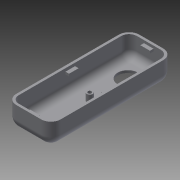
# Autodesk Inventor part: NodeMCU_MQ-7_top_shelled
Saved by Autodesk Inventor 2014 SP1 (Build 180222100, 222)
## iProperties
Created: 2016-10-27
Part Number: NodeMCU_MQ-7_top_shelled
Material: Generic
Document SubType Name: Modeling
Designer: danielsikar
Density: 1 g/cm^3
Appearance: Default
Author: danielsikar
Autodesk Inventor part; units mm, degrees
ref_plane "YZ Plane" through (0, 0, 0) normal (1, 0, 0) x (0, 1, 0)
ref_plane "XZ Plane" through (0, 0, 0) normal (0, 1, 0) x (-1, 0, 0)
ref_plane "XY Plane" through (0, 0, 0) normal (0, 0, 1) x (1, 0, 0)
sketch "Sketch1" plane through (0, 0, 0) normal (0, 0, 1) x (1, 0, 0)
  line L0 (0, 0) -> (37, 0)
  line L1 (37, 0) -> (37, 93.8)
  line L2 (28.5, 102.3) -> (8.5, 102.3)
  line L3 (0, 93.8) -> (0, 0)
  arc A0 (8.5, 102.3) -> (0, 93.8) centre (8.5, 93.8) ccw
  arc A1 (37, 93.8) -> (28.5, 102.3) centre (28.5, 93.8) ccw
  point P0 (37, 102.3)
  point P1 (0, 102.3)
  dimension "d0" = 37
  dimension "d1" = 102.3
  dimension "d11" = 8.5
  dimension "d12" = 8.5
  constraints: 8 end point, 4 point on circle, 4 point on line, 4 tangent, 2 centre point, 2 parallel, 1 horizontal, 1 perpendicular
  measures "d0" distance of point (0, 102.3) point (37, 102.3)
  measures "d1" distance of point (37, 102.3) L0.end
  measures "d11" radius of A0
  measures "d12" radius of A1
extrude "Extrusion1" add sketch "Sketch1" along normal blind 19
fillet "Fillet1" radius 8 2 edges at (0, 0, 9.5) (37, 0, 9.5)
fillet "Fillet2" radius 8 6 edges at (18.5, 102.3, 0) (0, 50.9, 0) (2.3431, 2.3431, 0) (18.5, 0, 0) (34.6569, 2.3431, 0) (37, 50.9, 0)
shell "Shell1" thickness 2 removed faces 1 at (12.3333, 36.6, 19)
sketch "Sketch2" plane through (0, 0, 0) normal (0, 0, -1) x (-1, 0, 0)
  circle A0 centre (-18.5, 82.8) radius 8.5
  line L0 (-8.5, 102.3) -> (-28.5, 102.3) projected
  point P0 (0, 0)
  point P1 (-8, 102.3)
  point P2 (-29, 102.3)
  dimension "d7" = 17
  dimension "d8" = 19.5
  constraints: 1 centre point
  measures "d7" diameter of A0
  measures "d8" distance from line of A0.centre L0
extrude "Extrusion2" cut sketch "Sketch2" against normal blind 19
sketch "Sketch3" plane through (8, 2, 8) normal (0, 1, 0) x (1, 0, 0)
  line L0 (21, -11) -> (0, -11) projected
  line L1 (6.6, -6.5) -> (14.6, -6.5)
  line L2 (14.6, -6.5) -> (14.6, -8.5)
  line L3 (14.6, -8.5) -> (6.6, -8.5)
  line L4 (6.6, -8.5) -> (6.6, -6.5)
  point P0 (-8, 8)
  point P1 (29, -11)
  dimension "d13" = 8
  dimension "d14" = 2
  dimension "d15" = 2.5
  dimension "d16" = 14.4
  constraints: 8 end point, 2 parallel, 1 horizontal, 1 perpendicular
  measures "d13" distance of L2.end L3.end
  measures "d14" distance of L1.end L2.end
  measures "d15" distance between parallel lines of L3 L0
  measures "d16" distance from line of point (29, -11) L2
extrude "Extrusion3" add sketch "Sketch3" along normal blind 3
sketch "Sketch4" plane through (2, 8, 8) normal (1, 0, 0) x (0, 0, -1)
  line L0 (-11, 0) -> (-11, 85.8) projected
  line L1 (-8.5, 47.15) -> (-6.5, 47.15)
  line L2 (-6.5, 47.15) -> (-6.5, 39.15)
  line L3 (-6.5, 39.15) -> (-8.5, 39.15)
  line L4 (-8.5, 39.15) -> (-8.5, 47.15)
  point P0 (8, -8)
  point P1 (-11, 94.3)
  dimension "d19" = 2
  dimension "d20" = 8
  dimension "d21" = 2.5
  dimension "d24" = 47.15
  constraints: 8 end point, 2 parallel, 1 horizontal, 1 perpendicular
  measures "d19" distance of L2.end L3.end
  measures "d20" distance of L1.end L2.end
  measures "d21" distance between parallel lines of L4 L0
  measures "d24" distance from line of point (-11, 94.3) L1
extrude "Extrusion4" add sketch "Sketch4" along normal blind 3
sketch "Sketch5" plane through (35, 8, 8) normal (-1, 0, 0) x (0, 0, 1)
  line L0 (11, 85.8) -> (11, 0) projected
  line L1 (6.5, 47.15) -> (8.5, 47.15)
  line L2 (8.5, 47.15) -> (8.5, 39.15)
  line L3 (8.5, 39.15) -> (6.5, 39.15)
  line L4 (6.5, 39.15) -> (6.5, 47.15)
  point P0 (-8, -8)
  point P1 (11, 94.3)
  dimension "d25" = 2
  dimension "d26" = 8
  dimension "d27" = 2.5
  dimension "d30" = 47.15
  constraints: 8 end point, 2 parallel, 1 horizontal, 1 perpendicular
  measures "d25" distance of L2.end L3.end
  measures "d26" distance of L1.end L2.end
  measures "d27" distance between parallel lines of L0 L2
  measures "d30" distance from line of point (11, 94.3) L1
extrude "Extrusion5" add sketch "Sketch5" along normal blind 3
sketch "Sketch6" plane through (8.5, 100.3, 8) normal (0, -1, 0) x (1, 0, 0)
  line L0 (5.9, 8.7641) -> (13.9, 8.7641)
  line L1 (13.9, 8.7641) -> (13.9, 6.7641)
  line L2 (13.9, 6.7641) -> (5.9, 6.7641)
  line L3 (5.9, 6.7641) -> (5.9, 8.7641)
  point P0 (-8.5, -8)
  point P1 (-8.5, 11)
  dimension "d31" = 8
  dimension "d32" = 2
  dimension "d33" = 14.4
  constraints: 8 end point, 2 parallel, 1 horizontal, 1 perpendicular
  measures "d31" distance of L1.end L2.end
  measures "d32" distance of L0.end L1.end
  measures "d33" distance from line of L3 point (-8.5, 11)
extrude "Extrusion6" add sketch "Sketch6" along normal blind 3
sketch "Sketch7" plane through (8, 8, 2) normal (0, 0, 1) x (1, 0, 0)
  circle A0 centre (10.5, 42.9) radius 1.5
  circle A1 centre (10.5, 42.9) radius 2.5
  point P0 (-8, -8)
  dimension "d36" = 3
  dimension "d37" = 5
  constraints: 2 centre point, 1 coincident
  measures "d36" diameter of A0
  measures "d37" diameter of A1
extrude "Extrusion7" add sketch "Sketch7" along normal blind 6
body "Solid1"
